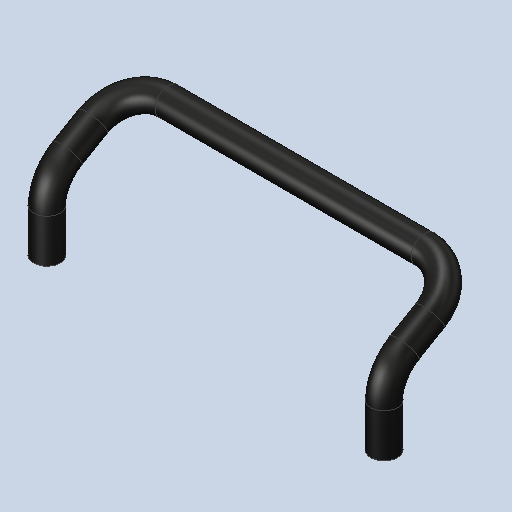
# Autodesk Inventor part: UHFNB125
Saved by Autodesk Inventor 2024.2 (Build 282272000, 272)
## iProperties
Category: PARTsolutions
Company: MISUMI
Created: 2024-01-05
Part Number: UHFNB125
Material: Aluminum 2014-T4
Catalog Web Link: https://jp.misumi-ec.com/vona2/detail/110300521620/?ProductCode=UHFNB125
Description: UHFN, UHFNS, UHFNA, UHFNEA, UHFNB, UHFNZ, UHFNSZ, UHFNAZ, UHFNEAZ, UHFNBZ_handle-Handles - Angle Type
Vendor: MISUMI
Document SubType Name: Modeling
Designer: psAdmin
Manufacturer: MISUMI
Mass: 48.8288 g
Surface Area: 77.0871 cm^2
Volume: 17.4389 cm^3
Density: 2.8 g/cm^3
Appearance: Glossy - Black
PSOL_IDENT_0: {$CADENAS_DATA/23d-libs/misumi/metric/43_levers_knobs/parts_uhfn/uhfn.prj},247 {VTYP=3D},{NB=UHFNB12
PSOL_IDENT_1: 5_h},{LINA=UHFNB125},{NN=UHFN, UHFNS, UHFNA, UHFNEA, UHFNB, UHFNZ, UHFNSZ, UHFNAZ, UHFNEAZ, UHFNBZ_h
PSOL_IDENT_2: andle},{DATE=04.06.2021 08:39:31},{GEOMDATE=30.04.2020 08:56:35},{VERSION=},{LINEID=120},{WBVAR=TS,M
PSOL_IDENT_3: AT,ST,MATW},{WBNUMERIC=}  {NB=UHFNB125_h},{LINA=UHFNB125},{KT=DUMMY},{PN=UHFNB125},{TYPE=UHFNB},{TS=
PSOL_IDENT_4: },{MAT=3},{ST=4},{MATW=},{ST1= '2', 'Buffing', '3', 'Alumite (Clear)','4', 'Electrostatic Coating (M
PSOL_IDENT_5: at Black)' },{L=125},{L1=135},{AL=2000},{MASS=136},{COLOR=0.00,0.00,0.00,0.00},{TS1='','w/o Washer','
PSOL_IDENT_6: Z','With Washer'},{MATW1='','N/A'},{X=9.50962},{Y=16.01924},{R=10.98076}
NB: UHFNB125_h
NN: UHFN, UHFNS, UHFNA, UHFNEA, UHFNB, UHFNZ, UHFNSZ, UHFNAZ, UHFNEAZ, UHFNBZ_handle
NT: Handles - Angle Type
NBSYN: $PN._h
LINA: UHFNB125
CATALOG: Misumi
PN: UHFNB125
TS: w/o  Washer
MAT: Aluminum Alloy
ST: Electrostatic Coating (Mat Black)
MATW: N/A
L: 125
L1: 135
AL: 2000
MASS: 136
SUPPLIER: MISUMI
ARTICLENO: UHFNB125_h
BOMINFO: UHFNB125
CREATOR: CADENAS GmbH
Title: UHFNB125
Author: Cadenas PARTsolutions
Comments: Handles - Angle Type
Autodesk Inventor part; units mm, degrees
sketch "_____1" plane through (0, 0, 0) normal (0, 1, 0) x (1, 0, 0)
  circle A0 centre (0, 0) radius 5
  constraints: 1 centre point
extrude "Extrusion1" add sketch "_____1" along normal blind 16.0192
sketch "_____2" plane through (0, 16.0192, 0) normal (0, 1, 0) x (1, 0, 0)
  line L0 (-50, 15) -> (50, 15)
  circle A0 centre (0, 0) radius 5
  constraints: 2 end point, 1 centre point
revolve "Revolution1" add sketch "_____2" angle 60 about axis through (-50, 16.0192, -15) along (-1, 0, 0)
sketch "_____3" plane through (0, 29.0096, -7.5) normal (0, 0.5, -0.8660254) x (1, 0, 0)
  circle A0 centre (0, 0) radius 5
  constraints: 1 centre point
extrude "Extrusion2" add sketch "_____3" along normal blind 10.9808
sketch "_____4" plane through (0, 34.5, -17.0096) normal (0, 0.5, -0.8660254) x (1, 0, 0)
  line L0 (15, 50) -> (15, -50)
  circle A0 centre (0, 0) radius 5
  constraints: 2 end point, 1 centre point
revolve "Revolution2" add sketch "_____4" angle 90 about axis through (15, -8.8013, -42.0096) along (0, -0.8660254, -0.5)
sketch "_____5" plane through (15, 42, -30) normal (1, 0, 0) x (0, -0.5, 0.8660254)
  circle A0 centre (0, 0) radius 5
  constraints: 1 centre point
extrude "Extrusion3" add sketch "_____5" along normal blind 95
sketch "_____6" plane through (110, 42, -30) normal (1, 0, 0) x (0, -0.5, 0.8660254)
  line L0 (15, 50) -> (15, -50)
  circle A0 centre (0, 0) radius 5
  constraints: 2 end point, 1 centre point
revolve "Revolution3" add sketch "_____6" angle 90 about axis through (110, -8.8013, -42.0096) along (0, -0.8660254, -0.5)
sketch "_____7" plane through (125, 34.5, -17.0096) normal (0, -0.5, 0.8660254) x (-1, 0, 0)
  circle A0 centre (0, 0) radius 5
  constraints: 1 centre point
extrude "Extrusion4" add sketch "_____7" along normal blind 10.9808
sketch "_____8" plane through (125, 29.0096, -7.5) normal (0, -0.5, 0.8660254) x (-1, 0, 0)
  line L0 (-50, 15) -> (50, 15)
  circle A0 centre (0, 0) radius 5
  constraints: 2 end point, 1 centre point
revolve "Revolution4" add sketch "_____8" angle 60 about axis through (175, 16.0192, -15) along (1, 0, 0)
sketch "_____9" plane through (125, 16.0192, 0) normal (0, -1, 0) x (-1, 0, 0)
  circle A0 centre (0, 0) radius 5
  constraints: 1 centre point
extrude "Extrusion5" add sketch "_____9" along normal blind 16.0192
sketch "Sketch10" plane through (0, 0, 0) normal (0, -1, 0) x (1, 0, 0)
  point P0 (0, 0)
hole "Hole1" at (0, 0, 0) direction (0, 1, 0) diameter 4.134 depth 15.6 tip angle 120 countersink diameter 5 countersink angle 90 thread size "M5x0.8" class "6H" standard "ISO Metric profile"
sketch "Sketch11" plane through (125, 0, 0) normal (0, -1, 0) x (1, 0, 0)
  point P0 (0, 0)
hole "Hole2" at (125, 0, 0) direction (0, 1, 0) diameter 4.134 depth 15.6 tip angle 120 countersink diameter 5 countersink angle 90 thread size "M5x0.8" class "6H" standard "ISO Metric profile"
ref_plane "H1_XY" through (0, 0, 0) normal (0, 1, 0) x (1, 0, 0)
ref_plane "H1_YZ" through (0, 0, 0) normal (1, 0, 0) x (0, 0, -1)
ref_plane "H1_ZX" through (0, 0, 0) normal (0, 0, -1) x (0, 1, 0)
ref_plane "H2_XY" through (125, 0, 0) normal (0, 1, 0) x (1, 0, 0)
ref_plane "H2_YZ" through (125, 0, 0) normal (1, 0, 0) x (0, 0, -1)
ref_plane "H2_ZX" through (125, 0, 0) normal (0, 0, -1) x (0, 1, 0)
body "Solid1"
